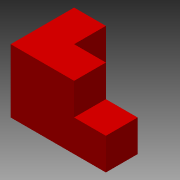
# Autodesk Inventor part: Part4
Saved by Autodesk Inventor 2013 (Build 170138000, 138)
## iProperties
Created: 2013-11-13
Part Number: Part4
Material: Generic
Document SubType Name: Modeling
Designer: s601298
Density: 1 g/cm^3
Author: s601298
Autodesk Inventor part; units mm, degrees
ref_plane "YZ Plane" through (0, 0, 0) normal (1, 0, 0) x (0, 1, 0)
ref_plane "XZ Plane" through (0, 0, 0) normal (0, 1, 0) x (-1, 0, 0)
ref_plane "XY Plane" through (0, 0, 0) normal (0, 0, 1) x (1, 0, 0)
sketch "Sketch1" plane through (0, 0, 0) normal (0, 1, 0) x (-1, 0, 0)
  line L0 (12.7594, -3.7732) -> (-44.3906, -3.7732)
  line L1 (-44.3906, -3.7732) -> (-44.3906, 15.2768)
  line L2 (-44.3906, 15.2768) -> (12.7594, 15.2768)
  line L3 (12.7594, 15.2768) -> (12.7594, -3.7732)
  point P0 (0, 0)
  dimension "d0" = 57.15
  dimension "d1" = 19.05
  constraints: 8 end point, 2 parallel, 1 horizontal, 1 perpendicular
  measures "d0" distance of L1.end L2.end
  measures "d1" distance of L0.end L1.end
extrude "Extrusion1" add sketch "Sketch1" along normal blind 19.05
sketch "Sketch2" plane through (0, 19.05, 0) normal (0, 1, 0) x (1, 0, 0)
  line L0 (-12.7594, 3.7732) -> (25.3406, 3.7732)
  line L1 (25.3406, 3.7732) -> (25.3406, -15.2768)
  line L2 (25.3406, -15.2768) -> (-12.7594, -15.2768)
  line L3 (-12.7594, -15.2768) -> (-12.7594, 3.7732)
  point P0 (0, 0)
  dimension "d4" = 38.1
  dimension "d5" = 19.05
  constraints: 8 end point, 2 parallel, 1 horizontal, 1 perpendicular
  measures "d4" distance of L1.end L2.end
  measures "d5" distance of L0.end L1.end
extrude "Extrusion2" add sketch "Sketch2" along normal blind 19.05
sketch "Sketch3" plane through (44.3906, 0, -3.7732) normal (0, 0, -1) x (-1, 0, 0)
  line L0 (57.15, 38.1) -> (38.1, 38.1)
  line L1 (38.1, 38.1) -> (38.1, 19.05)
  line L2 (38.1, 19.05) -> (57.15, 19.05)
  line L3 (57.15, 19.05) -> (57.15, 38.1)
  point P0 (44.3906, 0)
  dimension "d8" = 19.05
  dimension "d9" = 19.05
  constraints: 8 end point, 2 parallel, 1 horizontal, 1 perpendicular
  measures "d8" distance of L2.end L1.end
  measures "d9" distance of L1.end L0.end
extrude "Extrusion3" add sketch "Sketch3" along normal blind 19.05
body "Solid1"
